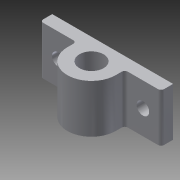
# Autodesk Inventor part: Shaft Mount V1.500 Drivetrain
Saved by Autodesk Inventor 2013 (Build 170138000, 138)
## iProperties
Created: 2013-01-06
Part Number: Shaft Mount V1.500 Drivetrain
Material: Aluminum 6061
Document SubType Name: Modeling
Designer: Moses
Density: 2.71 g/cm^3
Mass: 43.623 g
Surface Area: 65.3097 cm^2
Volume: 16.0971 cm^3
Author: Moses
Autodesk Inventor part; units mm, degrees
ref_plane "YZ Plane" through (0, 0, 0) normal (1, 0, 0) x (0, 1, 0)
ref_plane "XZ Plane" through (0, 0, 0) normal (0, 1, 0) x (-1, 0, 0)
ref_plane "XY Plane" through (0, 0, 0) normal (0, 0, 1) x (1, 0, 0)
sketch "Sketch1" plane through (0, 0, 0) normal (0, 1, 0) x (-1, 0, 0)
  line L0 (0, 0) -> (25.4, 0)
  line L1 (25.4, 0) -> (25.4, 23.8125)
  line L2 (25.4, 23.8125) -> (0, 23.8125)
  line L3 (0, 23.8125) -> (0, 0)
  circle A0 centre (12.7, 11.1125) radius 6.35
  line L4 (12.7, 23.8125) -> (12.7, 0) construction
  line L5 (-19.05, 6.35) -> (-19.05, 0)
  line L6 (-19.05, 0) -> (0, 0)
  line L7 (44.45, 6.35) -> (44.45, 0)
  line L8 (44.45, 0) -> (25.4, 0)
  line L9 (-19.05, 6.35) -> (0, 6.35)
  line L10 (25.4, 6.35) -> (44.45, 6.35)
  dimension "d0" = 25.4
  dimension "d1" = 23.8125
  dimension "d2" = 12.7
  dimension "d9" = 6.35
  dimension "d10" = 19.05
  dimension "d11" = 19.05
  dimension "d12" = 6.35
  dimension "d20" = 11.1125
  constraints: 22 end point, 5 parallel, 3 point on line, 2 horizontal, 2 midpoint, 1 centre point, 1 collinear, 1 perpendicular, 1 vertical
  measures "d0" distance of L2.end L1.end
  measures "d1" distance of L1.end L0.end
  measures "d2" diameter of A0
  measures "d9" distance of L5.start L5.end
  measures "d10" distance of L5.end L0.start
  measures "d11" distance of L7.end L0.end
  measures "d12" distance of L7.start L7.end
  measures "d20" distance from line of L0 A0.centre
extrude "Extrusion1" add sketch "Sketch1" along normal blind 25.4
fillet "Fillet1" radius 12.7 2 edges at (-25.4, 12.7, 23.8125) (0, 12.7, 23.8125)
fillet "Fillet1" radius 1.5875 4 edges at (-25.4, 12.7, 6.35) (0, 12.7, 6.35) (-44.45, 12.7, 6.35) (19.05, 12.7, 6.35)
sketch "Sketch2" plane through (19.05, 25.4, 0) normal (0, 0, -1) x (-1, 0, 0)
  line L0 (1.5875, 0) -> (1.5875, -25.4) construction
  line L1 (17.4625, 0) -> (1.5875, 0) construction
  line L2 (17.4625, -25.4) -> (17.4625, 0) construction
  line L3 (61.9125, -25.4) -> (61.9125, 0) construction
  line L4 (46.0375, 0) -> (46.0375, -25.4) construction
  line L5 (61.9125, 0) -> (46.0375, 0) construction
  line L6 (1.5875, -12.7) -> (17.4625, -12.7) construction
  line L7 (46.0375, -12.7) -> (61.9125, -12.7) construction
  circle A0 centre (9.525, -12.7) radius 3.302
  circle A1 centre (53.975, -12.7) radius 3.302
  line L8 (61.9125, -25.4) -> (46.0375, -25.4) projected
  line L9 (17.4625, -25.4) -> (1.5875, -25.4) projected
  point P0 (19.05, -25.4)
  dimension "d15" = 6.604
  dimension "d16" = 6.604
  dimension "d21" = 44.45
  constraints: 6 midpoint, 4 end point, 2 centre point
  measures "d15" diameter of A0
  measures "d16" diameter of A1
  measures "d21" distance of A1.centre A0.centre
extrude "Extrusion3" cut sketch "Sketch2" against normal through all
equation "\"d9\" = d12"
equation "\"d10\" = d11"
equation "\"d16\" = d15"
body "Solid1"
